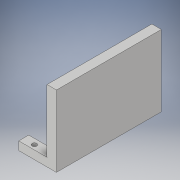
# Autodesk Inventor part: 000.705 - Пассивный прижим
Saved by Autodesk Inventor 2019 (Build 230136000, 136)
## iProperties
Created: 2020-02-29
Part Number: 000.705 - Пассивный прижим
Material: Типовые
Document SubType Name: Modeling
Designer: Петров Иван
Density: 1 g/cm^3
Appearance: По умолчанию
Author: Петров Иван
Autodesk Inventor part; units mm, degrees
ref_plane "YZ Plane" through (0, 0, 0) normal (1, 0, 0) x (0, 1, 0)
ref_plane "XZ Plane" through (0, 0, 0) normal (0, 1, 0) x (-1, 0, 0)
ref_plane "XY Plane" through (0, 0, 0) normal (0, 0, 1) x (1, 0, 0)
sketch "Эскиз1" plane through (0, 0, 0) normal (0, 1, 0) x (-1, 0, 0)
  line L0 (0, 0) -> (0, -20)
  circle A0 centre (0, -20) radius 2
  line L1 (-3.5, 25) -> (3.5, 25)
  line L2 (3.5, 25) -> (3.5, -25)
  line L3 (3.5, -25) -> (-3.5, -25)
  line L4 (-3.5, -25) -> (-3.5, 25)
  line L5 (-3.5, 25) -> (3.5, -25) construction
  line L6 (3.5, 25) -> (-3.5, -25) construction
  line L7 (0, 0) -> (0, 20)
  circle A1 centre (0, 20) radius 2
  dimension "d0" = 20
  dimension "d1" = 4
  dimension "d2" = 7
  dimension "d3" = 50
  dimension "d4" = 20
  dimension "d5" = 4
  constraints: 16 end point, 2 centre point, 2 coincident, 2 midpoint, 2 parallel, 1 horizontal, 1 perpendicular, 1 point on line, 1 vertical
  measures "d0" distance of L0.start L0.end
  measures "d1" diameter of A0
  measures "d2" distance of L2.end L3.end
  measures "d3" distance of L1.end L2.end
  measures "d4" distance of L0.start L7.end
  measures "d5" diameter of A1
extrude "Выдавливание1" add sketch "Эскиз1" along normal blind 4 contours A0 | L1 L2 L3 L4 | A1
sketch "Эскиз2" plane through (3.5, 0, 25) normal (1, 0, 0) x (0, 0, -1)
  line L0 (50, 0) -> (0, 0) projected
  line L1 (0, 4) -> (50, 4)
  line L2 (50, 4) -> (50, 0)
  line L3 (50, 0) -> (0, 0)
  line L4 (0, 0) -> (0, 4)
  point P0 (25, 0)
  constraints: 8 end point, 2 parallel, 1 horizontal, 1 perpendicular
extrude "Выдавливание2" add sketch "Эскиз2" along normal blind 7
sketch "Эскиз3" plane through (0, 4, 0) normal (0, 1, 0) x (1, 0, 0)
  line L0 (-3.5, -25) -> (10.5, -25) projected
  line L1 (-3.5, 25) -> (10.5, 25) projected
  line L2 (10.5, -25) -> (3.5, -25)
  line L3 (3.5, -25) -> (3.5, 25)
  line L4 (3.5, 25) -> (10.5, 25)
  line L5 (10.5, 25) -> (10.5, -25)
  point P0 (0, 0)
  dimension "d10" = 7
  constraints: 8 end point, 2 parallel, 1 horizontal, 1 midpoint, 1 perpendicular
  measures "d10" distance of L3.end L4.end
extrude "Выдавливание3" add sketch "Эскиз3" along normal blind 30
sketch "Эскиз5" plane through (0, 4, 0) normal (0, 1, 0) x (1, 0, 0)
  line L0 (-7.5352, -8.6362) -> (-7.5352, -8.5162)
  arc A0 (-1.7352, -8.5162) -> (-7.5352, -8.5162) centre (-4.6352, -8.5162) ccw
  line L1 (-1.7352, -8.5162) -> (-1.7352, -8.6362)
  arc A1 (1.3648, -12.5541) -> (-1.7352, -8.6362) centre (-4.6352, -14.1162) ccw
  line L2 (1.3648, -12.5541) -> (1.3648, 1.4338)
  arc A2 (1.3648, 1.4338) -> (0.6148, 2.1838) centre (0.6148, 1.4338) ccw
  line L3 (0.6148, 2.1838) -> (-9.8852, 2.1838)
  arc A3 (-9.8852, 2.1838) -> (-10.6352, 1.4338) centre (-9.8852, 1.4338) ccw
  line L4 (-10.6352, 1.4338) -> (-10.6352, -12.5541)
  arc A4 (-7.5352, -8.6362) -> (-10.6352, -12.5541) centre (-4.6352, -14.1162) ccw
  line L5 (0.4648, -4.2162) -> (0.4648, 0.7838)
  arc A5 (-0.0352, -4.7162) -> (0.4648, -4.2162) centre (-0.0352, -4.2162) ccw
  line L6 (-9.2352, -4.7162) -> (-0.0352, -4.7162)
  arc A6 (-9.7352, -4.2162) -> (-9.2352, -4.7162) centre (-9.2352, -4.2162) ccw
  line L7 (-9.7352, 0.7838) -> (-9.7352, -4.2162)
  arc A7 (-9.2352, 1.2838) -> (-9.7352, 0.7838) centre (-9.2352, 0.7838) ccw
  line L8 (-0.0352, 1.2838) -> (-9.2352, 1.2838)
  arc A8 (0.4648, 0.7838) -> (-0.0352, 1.2838) centre (-0.0352, 0.7838) ccw
  arc A9 (-5.1852, 5.8865) -> (-4.0852, 5.8865) centre (-4.6352, 4.9338) ccw
  line L9 (-5.1852, 7.0838) -> (-5.1852, 5.8865)
  line L10 (-5.1852, 7.0838) -> (-9.8852, 7.0838)
  arc A10 (-9.8852, 7.0838) -> (-10.7352, 6.2338) centre (-9.8852, 6.2338) ccw
  line L11 (-10.7352, 6.2338) -> (-10.7352, 1.4338)
  arc A11 (-9.8852, 2.2838) -> (-10.7352, 1.4338) centre (-9.8852, 1.4338) ccw
  line L12 (0.6148, 2.2838) -> (-9.8852, 2.2838)
  arc A12 (1.4648, 1.4338) -> (0.6148, 2.2838) centre (0.6148, 1.4338) ccw
  line L13 (1.4648, 1.4338) -> (1.4648, 6.2338)
  arc A13 (1.4648, 6.2338) -> (0.6148, 7.0838) centre (0.6148, 6.2338) ccw
  line L14 (0.6148, 7.0838) -> (-4.0852, 7.0838)
  line L15 (-4.0852, 5.8865) -> (-4.0852, 7.0838)
  line L16 (-9.8852, -25.0162) -> (-5.1852, -25.0162)
  line L17 (-5.1852, -23.8188) -> (-5.1852, -25.0162)
  arc A14 (-4.0852, -23.8188) -> (-5.1852, -23.8188) centre (-4.6352, -22.8662) ccw
  line L18 (-4.0852, -25.0162) -> (-4.0852, -23.8188)
  line L19 (-4.0852, -25.0162) -> (0.6148, -25.0162)
  arc A15 (0.6148, -25.0162) -> (1.4648, -24.1662) centre (0.6148, -24.1662) ccw
  line L20 (1.4648, -24.1662) -> (1.4648, -19.3662)
  arc A16 (0.6148, -20.2162) -> (1.4648, -19.3662) centre (0.6148, -19.3662) ccw
  line L21 (-9.8852, -20.2162) -> (0.6148, -20.2162)
  arc A17 (-10.7352, -19.3662) -> (-9.8852, -20.2162) centre (-9.8852, -19.3662) ccw
  line L22 (-10.7352, -19.3662) -> (-10.7352, -24.1662)
  arc A18 (-10.7352, -24.1662) -> (-9.8852, -25.0162) centre (-9.8852, -24.1662) ccw
  line L23 (-10.7352, -19.3662) -> (-10.7352, -15.6782)
  line L24 (-10.7352, -12.5541) -> (-10.7352, -14.1162)
  line L25 (-10.7352, -14.1162) -> (-10.7352, -15.6782)
  line L26 (-10.7352, -12.5541) -> (-10.7352, 1.4338)
  line L27 (1.4648, 1.4338) -> (1.4648, -12.5541)
  line L28 (1.4648, -15.6782) -> (1.4648, -19.3662)
  line L29 (1.4648, -15.6782) -> (1.4648, -14.1162)
  line L30 (1.4648, -14.1162) -> (1.4648, -12.5541)
  arc A19 (-10.6352, -15.6782) -> (-6.1972, -20.1162) centre (-4.6352, -14.1162) ccw
  line L31 (-10.6352, -15.6782) -> (-10.6352, -19.3662)
  arc A20 (-10.6352, -19.3662) -> (-9.8852, -20.1162) centre (-9.8852, -19.3662) ccw
  line L32 (-9.8852, -20.1162) -> (-6.1972, -20.1162)
  line L33 (1.3648, -19.3662) -> (1.3648, -15.6782)
  arc A21 (-3.0731, -20.1162) -> (1.3648, -15.6782) centre (-4.6352, -14.1162) ccw
  line L34 (-3.0731, -20.1162) -> (0.6148, -20.1162)
  arc A22 (0.6148, -20.1162) -> (1.3648, -19.3662) centre (0.6148, -19.3662) ccw
  circle A23 centre (-4.6352, 4.9338) radius 1.1
  line L35 (-5.1852, 5.8865) -> (-5.1852, 7.0838)
  line L36 (-4.0852, 7.0838) -> (-5.1852, 7.0838)
  circle A24 centre (-4.6352, -22.8662) radius 1.1
  line L37 (-5.1852, -25.0162) -> (-5.1852, -23.8188)
  line L38 (-4.0852, -25.0162) -> (-5.1852, -25.0162)
  circle A25 centre (-4.6352, -14.1162) radius 0.8
  line L39 (-3.5, 25) -> (3.5, 25) projected
  line L40 (-13.5, 25) -> (-13.5, -25)
  line L41 (-13.5, -25) -> (-3.5, -25)
  line L42 (-3.5, -25) -> (-3.5, 25)
  point P0 (0, 0)
  point P1 (-4.6352, -8.9662)
  dimension "d16" = 10
  constraints: 84 end point, 46 point on circle, 25 centre point, 2 coincident, 1 collinear, 1 concentric, 1 parallel, 3 other
  measures "d16" distance of L41.end L40.end
extrude "Выдавливание5" cut sketch "Эскиз5" against normal blind 10 contours A4 L4 A3 L3 L42 L8 A7 L7 A6 L6 A0 L0 | L0 A0 L42 L21 A17 L23 L25 L24 L26 A11 L12 L3 A3 L4 A4 | L42 L6 A5 L5 A8 L8 L3 A2 L2 A1 L1 A0 | A0 L1 A1 L2 A2 L3 L42 L12 A12 L27 L30 L29 L28 A16 L21 | L42 L8 A8 L5 A5 L6 | L6 A6 L7 A7 L8 L42 | A19 L32 A20 L31 | A22 L34 A21 L33 | A25
move faces "Перенос1" translate (-6.504, 0, 0) faces at (-3.5, 2.6667, -9.8559) (-3.5, 1.3333, 23.4054)
sketch "Эскиз6" plane through (0, 4, 0) normal (0, 1, 0) x (1, 0, 0)
  arc A0 (1.4648, -18.6645) -> (1.4648, -9.5679) centre (-2.6, -14.1162) ccw
  line L0 (1.4648, -9.5679) -> (1.4648, -19.3662)
  point P0 (0, 0)
  point P1 (0.2532, -8.7246)
  point P2 (-5.4532, -8.7246)
  constraints: 2 end point, 2 point on circle, 1 centre point, 1 point on line
extrude "Выдавливание6" cut sketch "Эскиз6" against normal blind 7
sketch "Эскиз7" plane through (0, 0, 0) normal (0, -1, 0) x (1, 0, 0)
  line L0 (-10.004, 25) -> (-10.004, 20.2162) projected
  line L1 (-10.004, 21.4561) -> (4.0826, 21.4561)
  line L2 (4.0826, 21.4561) -> (4.0826, -3.0396)
  line L3 (4.0826, -3.0396) -> (-10.004, -3.0396)
  line L4 (-10.004, -3.0396) -> (-10.004, 21.4561)
  point P0 (0, 0)
  constraints: 8 end point, 2 parallel, 1 horizontal, 1 perpendicular, 1 point on line
extrude "Выдавливание7" cut sketch "Эскиз7" against normal blind 0.3
sketch "Эскиз8" plane through (0, 4, 0) normal (0, 1, 0) x (1, 0, 0)
  line L0 (-7.5352, -8.6362) -> (-7.5352, -8.5162)
  arc A0 (-1.7352, -8.5162) -> (-7.5352, -8.5162) centre (-4.6352, -8.5162) ccw
  line L1 (-1.7352, -8.5162) -> (-1.7352, -8.6362)
  arc A1 (1.3648, -12.5541) -> (-1.7352, -8.6362) centre (-4.6352, -14.1162) ccw
  line L2 (1.3648, -12.5541) -> (1.3648, 1.4338)
  arc A2 (1.3648, 1.4338) -> (0.6148, 2.1838) centre (0.6148, 1.4338) ccw
  line L3 (0.6148, 2.1838) -> (-9.8852, 2.1838)
  arc A3 (-9.8852, 2.1838) -> (-10.6352, 1.4338) centre (-9.8852, 1.4338) ccw
  line L4 (-10.6352, 1.4338) -> (-10.6352, -12.5541)
  arc A4 (-7.5352, -8.6362) -> (-10.6352, -12.5541) centre (-4.6352, -14.1162) ccw
  line L5 (0.4648, -4.2162) -> (0.4648, 0.7838)
  arc A5 (-0.0352, -4.7162) -> (0.4648, -4.2162) centre (-0.0352, -4.2162) ccw
  line L6 (-9.2352, -4.7162) -> (-0.0352, -4.7162)
  arc A6 (-9.7352, -4.2162) -> (-9.2352, -4.7162) centre (-9.2352, -4.2162) ccw
  line L7 (-9.7352, 0.7838) -> (-9.7352, -4.2162)
  arc A7 (-9.2352, 1.2838) -> (-9.7352, 0.7838) centre (-9.2352, 0.7838) ccw
  line L8 (-0.0352, 1.2838) -> (-9.2352, 1.2838)
  arc A8 (0.4648, 0.7838) -> (-0.0352, 1.2838) centre (-0.0352, 0.7838) ccw
  arc A9 (-5.1852, 5.8865) -> (-4.0852, 5.8865) centre (-4.6352, 4.9338) ccw
  line L9 (-5.1852, 7.0838) -> (-5.1852, 5.8865)
  line L10 (-5.1852, 7.0838) -> (-9.8852, 7.0838)
  arc A10 (-9.8852, 7.0838) -> (-10.7352, 6.2338) centre (-9.8852, 6.2338) ccw
  line L11 (-10.7352, 6.2338) -> (-10.7352, 1.4338)
  arc A11 (-9.8852, 2.2838) -> (-10.7352, 1.4338) centre (-9.8852, 1.4338) ccw
  line L12 (0.6148, 2.2838) -> (-9.8852, 2.2838)
  arc A12 (1.4648, 1.4338) -> (0.6148, 2.2838) centre (0.6148, 1.4338) ccw
  line L13 (1.4648, 1.4338) -> (1.4648, 6.2338)
  arc A13 (1.4648, 6.2338) -> (0.6148, 7.0838) centre (0.6148, 6.2338) ccw
  line L14 (0.6148, 7.0838) -> (-4.0852, 7.0838)
  line L15 (-4.0852, 5.8865) -> (-4.0852, 7.0838)
  line L16 (-9.8852, -25.0162) -> (-5.1852, -25.0162)
  line L17 (-5.1852, -23.8188) -> (-5.1852, -25.0162)
  arc A14 (-4.0852, -23.8188) -> (-5.1852, -23.8188) centre (-4.6352, -22.8662) ccw
  line L18 (-4.0852, -25.0162) -> (-4.0852, -23.8188)
  line L19 (-4.0852, -25.0162) -> (0.6148, -25.0162)
  arc A15 (0.6148, -25.0162) -> (1.4648, -24.1662) centre (0.6148, -24.1662) ccw
  line L20 (1.4648, -24.1662) -> (1.4648, -19.3662)
  arc A16 (0.6148, -20.2162) -> (1.4648, -19.3662) centre (0.6148, -19.3662) ccw
  line L21 (-9.8852, -20.2162) -> (0.6148, -20.2162)
  arc A17 (-10.7352, -19.3662) -> (-9.8852, -20.2162) centre (-9.8852, -19.3662) ccw
  line L22 (-10.7352, -19.3662) -> (-10.7352, -24.1662)
  arc A18 (-10.7352, -24.1662) -> (-9.8852, -25.0162) centre (-9.8852, -24.1662) ccw
  line L23 (-10.7352, -19.3662) -> (-10.7352, -15.6782)
  line L24 (-10.7352, -12.5541) -> (-10.7352, -14.1162)
  line L25 (-10.7352, -14.1162) -> (-10.7352, -15.6782)
  line L26 (-10.7352, -12.5541) -> (-10.7352, 1.4338)
  line L27 (1.4648, 1.4338) -> (1.4648, -12.5541)
  line L28 (1.4648, -15.6782) -> (1.4648, -19.3662)
  line L29 (1.4648, -15.6782) -> (1.4648, -14.1162)
  line L30 (1.4648, -14.1162) -> (1.4648, -12.5541)
  arc A19 (-10.6352, -15.6782) -> (-6.1972, -20.1162) centre (-4.6352, -14.1162) ccw
  line L31 (-10.6352, -15.6782) -> (-10.6352, -19.3662)
  arc A20 (-10.6352, -19.3662) -> (-9.8852, -20.1162) centre (-9.8852, -19.3662) ccw
  line L32 (-9.8852, -20.1162) -> (-6.1972, -20.1162)
  line L33 (1.3648, -19.3662) -> (1.3648, -15.6782)
  arc A21 (-3.0731, -20.1162) -> (1.3648, -15.6782) centre (-4.6352, -14.1162) ccw
  line L34 (-3.0731, -20.1162) -> (0.6148, -20.1162)
  arc A22 (0.6148, -20.1162) -> (1.3648, -19.3662) centre (0.6148, -19.3662) ccw
  circle A23 centre (-4.6352, 4.9338) radius 1.1
  line L35 (-5.1852, 5.8865) -> (-5.1852, 7.0838)
  line L36 (-4.0852, 7.0838) -> (-5.1852, 7.0838)
  circle A24 centre (-4.6352, -22.8662) radius 1.1
  line L37 (-5.1852, -25.0162) -> (-5.1852, -23.8188)
  line L38 (-4.0852, -25.0162) -> (-5.1852, -25.0162)
  circle A25 centre (-4.6352, -14.1162) radius 0.8
  line L39 (-3.5, 25) -> (3.5, 25)
  line L40 (-13.5, 25) -> (-13.5, -25)
  line L41 (-13.5, -25) -> (-3.5, -25)
  line L42 (-3.5, -25) -> (-3.5, 25)
  point P0 (0, 0)
  point P1 (0, 0)
  point P2 (-4.6352, -8.9662)
  dimension "d26" = 10
  constraints: 86 end point, 46 point on circle, 25 centre point, 2 coincident, 1 collinear, 1 concentric, 1 parallel, 3 other
  measures "d26" distance of L41.end L40.end
extrude "Выдавливание8" cut sketch "Эскиз8" against normal through all contours A24 A14 | A9 A23
move faces "Перенос2" translate (-2.5, 0, 0) faces at (10.5, 11.3333, -8.3333)
